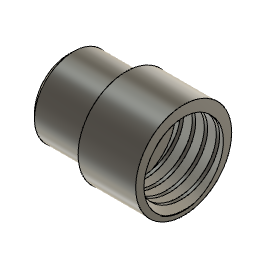
thread18F (Autodesk Fusion 360 design; units mm, degrees)
Autodesk Fusion 360 part; units mm, degrees
sketch "Sketch1" plane through (0, 0, 0) normal (1, 0, 0) x (0, 1, 0)
  circle A0 centre (0, 0) radius 8.1
  dimension "d1" = 16.2
  constraint coincident A0.centre origin
  measures "d1" diameter of A0
extrude "Extrude1" add sketch "Sketch1" against normal blind 12
sketch "Sketch2" plane through (0, 0, 0) normal (1, 0, 0) x (0, 1, 0)
  circle A0 centre (0, 0) radius 8.1
  circle A1 centre (0, 0) radius 10
  dimension "d4" = 20
  constraint coincident A0.centre A1.centre
  measures "d4" diameter of A1
extrude "Extrude2" add sketch "Sketch2" along normal blind 12 contours A0 | A1
chamfer "Chamfer1" distance 1.3 angle 45 1 edges at (0, -7.5519, -2.9291)
sketch "Sketch3" plane through (12, 0, 0) normal (1, 0, 0) x (0, 1, 0)
  circle A0 centre (0, 0) radius 10
  circle A1 centre (0, 0) radius 9
  dimension "d8" = 18
  constraint coincident A0.centre A1.centre
  measures "d8" diameter of A1
extrude "Extrude3" cut sketch "Sketch3" against normal blind 10 contours A1
thread "Thread1" "ISO Metric profile 18.0 M18x2.5 6H" major diameter 18.2926 minor diameter 15.5187 pitch 2.5 angle 60 modelled right hand crest width 0.6901 on face at (5.3333, 8.9888, -0.4486) crest through (11.375, 7.7594, 0)
chamfer "Chamfer2" distance 1 angle 45 1 edges at (-12, -7.5519, 2.9291)
